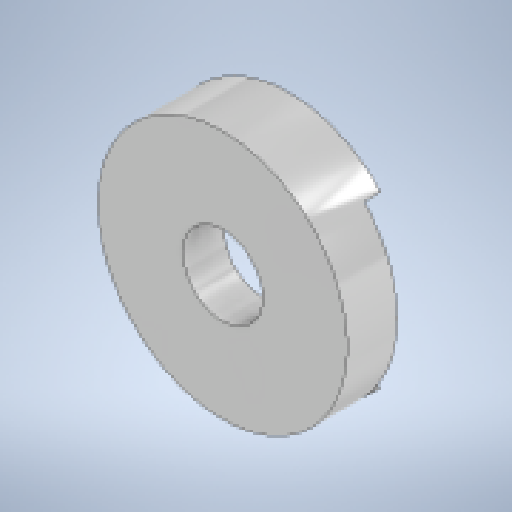
# Autodesk Inventor part: axis_4_top_frame
Saved by Autodesk Inventor 2024.1 (Build 281209000, 209)
## iProperties
Created: 2023-10-02
Part Number: axis_4_top_frame
Material: Aluminum 6061-AHC
Document SubType Name: Modeling
Designer: chanh
Density: 2.7 g/cm^3
Appearance: Aluminum - Dark
Author: chanh
Autodesk Inventor part; units mm, degrees
ref_plane "YZ Plane" through (0, 0, 0) normal (1, 0, 0) x (0, 1, 0)
ref_plane "XZ Plane" through (0, 0, 0) normal (0, 1, 0) x (-1, 0, 0)
ref_plane "XY Plane" through (0, 0, 0) normal (0, 0, 1) x (1, 0, 0)
sketch "Sketch8" plane through (0, 0, 0) normal (0, 0, 1) x (1, 0, 0)
  circle A0 centre (0, 0) radius 15
  dimension "d33" = 30
  constraints: 1 centre point, 1 coincident
  measures "d33" diameter of A0
extrude "Extrusion7" add sketch "Sketch8" against normal blind 8
sketch "Sketch10" plane through (0, 0, -8) normal (0, 0, -1) x (-1, 0, 0)
  line L0 (6, -10.07) -> (-26.1, -10.07)
  line L1 (6, -8.07) -> (6, -10.07)
  arc A0 (8, -6.07) -> (6, -8.07) centre (8, -8.07) ccw
  line L2 (10, -6.07) -> (8, -6.07)
  line L3 (10, 6.07) -> (10, -6.07)
  line L4 (8, 6.07) -> (10, 6.07)
  arc A1 (6, 8.07) -> (8, 6.07) centre (8, 8.07) ccw
  line L5 (6, 10.07) -> (6, 8.07)
  line L6 (-26.1, 10.07) -> (6, 10.07)
  line L7 (-26.1, 10.07) -> (-26.1, -10.07)
  line L8 (-26.2, -10.17) -> (6.1, -10.17)
  line L9 (6.1, -10.17) -> (6.1, -8.07)
  arc A2 (8, -6.17) -> (6.1, -8.07) centre (8, -8.07) ccw
  line L10 (8, -6.17) -> (10.1, -6.17)
  line L11 (10.1, -6.17) -> (10.1, 6.17)
  line L12 (10.1, 6.17) -> (8, 6.17)
  arc A3 (6.1, 8.07) -> (8, 6.17) centre (8, 8.07) ccw
  line L13 (6.1, 8.07) -> (6.1, 10.17)
  line L14 (6.1, 10.17) -> (-26.2, 10.17)
  line L15 (-26.2, 10.17) -> (-26.2, -10.17)
  point P0 (0, 0)
  dimension "d36" = 0.1
  constraints: 32 end point, 8 point on circle, 4 centre point, 4 horizontal, 4 vertical, 23 other
  measures "d36" distance between parallel lines of L0 L8
extrude "Extrusion8" cut sketch "Sketch10" against normal blind 2 contours L0 L7 L6 L5 A1 L4 L3 L2 A0 L1 | L15 L14 L13 A3 L12 L11 L10 A2 L9 L8
sketch "Sketch11" plane through (0, 0, -6) normal (0, 0, -1) x (-1, 0, 0)
  circle A0 centre (0, 0) radius 6.4
  point P0 (0, 0)
  constraints: 1 centre point, 2 other
extrude "Extrusion9" cut sketch "Sketch11" against normal blind 1.1
sketch "Sketch12" plane through (0, 0, -4.9) normal (0, 0, -1) x (-1, 0, 0)
  circle A0 centre (0, 0) radius 4.8
  dimension "d41" = 9.6
  constraints: 1 centre point, 1 coincident
  measures "d41" diameter of A0
extrude "Extrusion10" cut sketch "Sketch12" against normal blind 4.9
body "Solid2"
